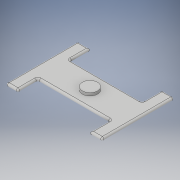
# Autodesk Inventor part: SujetorPanel
Saved by Autodesk Inventor 2019 (Build 230136000, 136)
## iProperties
Created: 2020-08-08
Part Number: SujetorPanel
Material: Generic
Document SubType Name: Modeling
Designer: Sergio
Density: 1 g/cm^3
Appearance: Default
Author: Sergio
Autodesk Inventor part; units mm, degrees
ref_plane "YZ Plane" through (0, 0, 0) normal (1, 0, 0) x (0, 1, 0)
ref_plane "XZ Plane" through (0, 0, 0) normal (0, 1, 0) x (-1, 0, 0)
ref_plane "XY Plane" through (0, 0, 0) normal (0, 0, 1) x (1, 0, 0)
sketch "Sketch1" plane through (0, 0, 0) normal (0, 1, 0) x (-1, 0, 0)
  line L0 (-45.5, -20) -> (45.5, -20)
  line L1 (60.5, -20) -> (60.5, 20)
  line L2 (45.5, 20) -> (-45.5, 20)
  line L3 (-60.5, 20) -> (-60.5, -20)
  line L4 (-60.5, -20) -> (60.5, 20) construction
  line L5 (60.5, -20) -> (-60.5, 20) construction
  line L6 (-60.5, -45) -> (60.5, -45) construction
  line L7 (60.5, -45) -> (60.5, 45) construction
  line L8 (60.5, 45) -> (-60.5, 45) construction
  line L9 (-60.5, 45) -> (-60.5, -45) construction
  line L10 (-60.5, -45) -> (60.5, 45) construction
  line L11 (60.5, -45) -> (-60.5, 45) construction
  line L12 (60.5, 45) -> (45.5, 45)
  line L13 (45.5, -45) -> (60.5, -45)
  line L14 (60.5, -45) -> (60.5, 45)
  line L15 (-60.5, -45) -> (-45.5, -45)
  line L16 (-45.5, 45) -> (-60.5, 45)
  line L17 (-60.5, 45) -> (-60.5, -45)
  line L18 (-45.5, -45) -> (-45.5, -20)
  line L19 (-45.5, 20) -> (-45.5, 45)
  line L20 (45.5, 45) -> (45.5, 20)
  line L21 (45.5, -20) -> (45.5, -45)
  point P0 (0, 0)
  dimension "d0" = 121
  dimension "d1" = 40
  dimension "d2" = 121
  dimension "d3" = 90
  dimension "d4" = 15
  dimension "d5" = 15
  constraints: 44 end point, 10 parallel, 6 perpendicular, 4 horizontal, 4 midpoint, 2 point on line
  measures "d0" distance of L3.start L1.end
  measures "d1" distance of L1.start L1.end
  measures "d2" distance of L8.end L7.end
  measures "d3" distance of L7.end L6.end
  measures "d4" distance of L13.end L13.start
  measures "d5" distance of L16.end L16.start
extrude "Extrusion1" add sketch "Sketch1" along normal blind 4
sketch "Sketch2" plane through (0, 4, 0) normal (0, 1, 0) x (1, 0, 0)
  circle A0 centre (0, 0) radius 9.5
  dimension "d8" = 19
  constraints: 1 centre point, 1 coincident
  measures "d8" diameter of A0
extrude "Extrusion2" add sketch "Sketch2" along normal blind 3.5
fillet "Fillet1" radius 2 22 edges at (-60.5, 0, 0) (-53, 0, -45) (-45.5, 0, -32.5) (0, 0, -20) (0, 0, 20) (45.5, 0, -32.5) (53, 0, -45) (60.5, 0, 0) (53, 0, 45) (45.5, 0, 32.5) (60.5, 2, 45) (60.5, 2, -45) (45.5, 2, -45) (45.5, 2, -20) (45.5, 2, 20) (-45.5, 2, 20) (-45.5, 2, -20) (-60.5, 2, -45) (-60.5, 2, 45) (-45.5, 2, 45) (-53, 0, 45) (-45.5, 0, 32.5)
fillet "Fillet2" radius 2 18 edges at (-59.9142, 4, -44.4142) (-60.5, 4, 0) (-59.9142, 4, 44.4142) (-53, 4, 45) (-46.0858, 4, 44.4142) (-45.5, 4, 32.5) (0, 4, 20) (45.5, 4, 33.5) (-52, 4, -45) (0, 4, -20) (45.5, 4, -32.5) (46.0858, 4, -44.4142) (53, 4, -45) (59.9142, 4, -44.4142) (60.5, 4, 0) (59.9142, 4, 44.4142) (52, 4, 45) (-45.5, 4, -33.5)
body "Solid1"
